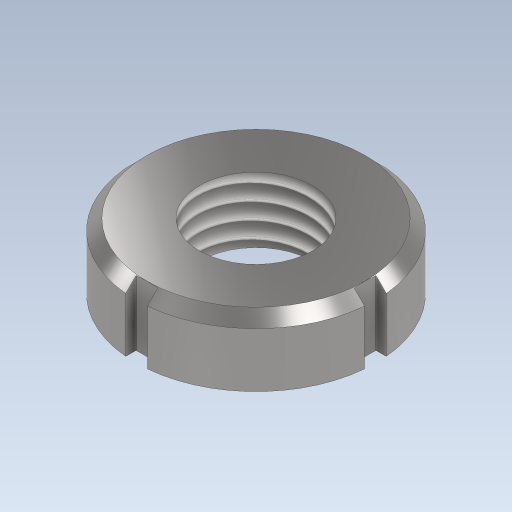
# Autodesk Inventor part: Pump-Motor-CW-Rotation:Lock Nut
Saved by Autodesk Inventor 2024.2 (Build 282272000, 272)
## iProperties
Created: 2025-06-16
Material: Stainless Steel
Document SubType Name: Modeling
Density: 8 g/cm^3
Appearance: Semi-Polished
Designer: cw
Author: cw
Autodesk Inventor part; units mm, degrees
ref_plane "YZ Plane" through (0, 0, 0) normal (1, 0, 0) x (0, 1, 0)
ref_plane "XZ Plane" through (0, 0, 0) normal (0, 1, 0) x (-1, 0, 0)
ref_plane "XY Plane" through (0, 0, 0) normal (0, 0, 1) x (1, 0, 0)
sketch "Sketch1" plane through (0, 0, 0) normal (0, 0, 1) x (1, 0, 0)
  circle A0 centre (0, 0) radius 11
  dimension "d0" = 22
  constraints: 1 centre point, 1 coincident
  measures "d0" diameter of A0
extrude "Extrusion1" add sketch "Sketch1" along normal mid plane 6
sketch "Sketch3" plane through (0, 0, 3) normal (0, 0, 1) x (1, 0, 0)
  point P0 (0, 0)
hole "Hole1" at (0, 0, 3) direction (0, 0, -1) diameter 10.376 end through all thread size "M12x1.5" class "6H" standard "ISO Metric profile"
sketch "Sketch2" plane through (0, 0, 3) normal (0, 0, 1) x (1, 0, 0)
  line L0 (11, 1) -> (10, 1)
  line L1 (10, 1) -> (10, -1)
  line L2 (10, -1) -> (11, -1)
  line L3 (11, -1) -> (11, 1)
  circle A0 centre (0, 0) radius 11 construction
  point P0 (10, 0)
  dimension "d3" = 2
  dimension "d4" = 1
  constraints: 8 end point, 2 parallel, 1 horizontal, 1 horizontal alignment, 1 midpoint, 1 perpendicular, 1 tangent
  measures "d3" distance of L2.end L0.start
  measures "d4" distance of L1.end L2.end
extrude "Extrusion2" cut sketch "Sketch2" against normal through all
pattern_circular "Circular Pattern1" count 4 over 360 about axis through (0, 0, 0) along (0, 0, 1) of "Extrusion2"
chamfer "Chamfer1" distance 1 angle 45 4 edges at (7.7782, -7.7782, 3) (7.7782, 7.7782, 3) (-7.7782, 7.7782, 3) (-7.7782, -7.7782, 3)
body "Solid1"
